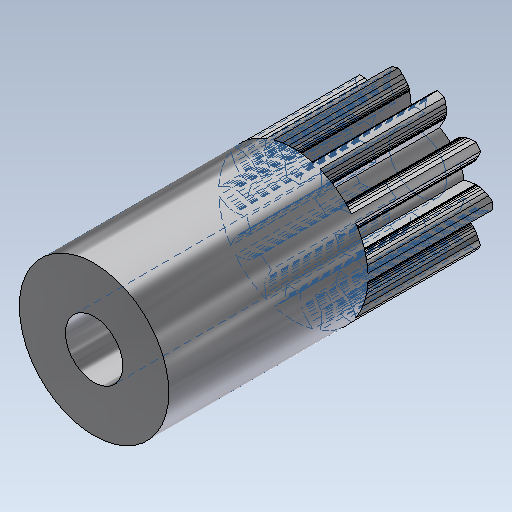
# Autodesk Inventor part: ピニオン10
Saved by Autodesk Inventor 2020 (Build 240168000, 168)
## iProperties
Created: 2015-02-03
Part Number: ピニオン10
Material: 鋼、炭素鋼
Document SubType Name: Modeling
Designer: Riku
Mass: 5 g
Surface Area: 4.55834 cm^2
Volume: 0.265293 cm^3
Density: 18.8471 g/cm^3
Appearance: 半つや出し
Author: Riku
Autodesk Inventor part; units mm, degrees
ref_plane "YZ Plane" through (0, 0, 0) normal (1, 0, 0) x (0, 1, 0)
ref_plane "XZ Plane" through (0, 0, 0) normal (0, 1, 0) x (-1, 0, 0)
ref_plane "XY Plane" through (0, 0, 0) normal (0, 0, 1) x (1, 0, 0)
sketch "スケッチ1" plane through (0, 0, 0) normal (0, 0, 1) x (1, 0, 0)
  arc A0 (148.8341, 107.332) -> (148.8329, 107.3255) centre (148.9303, 107.3099) ccw
  line L0 (148.8329, 107.3255) -> (148.7657, 106.8561)
  arc A1 (148.7657, 106.8561) -> (148.2343, 106.8561) centre (148.5, 105) ccw
  line L1 (148.2343, 106.8561) -> (148.1671, 107.3255)
  arc A2 (148.1671, 107.3255) -> (148.1659, 107.332) centre (148.0697, 107.3099) ccw
  arc A3 (148.1659, 107.332) -> (148.1608, 107.3513) centre (147.9057, 107.2734) ccw
  arc A4 (148.1608, 107.3513) -> (148.1495, 107.3837) centre (147.7349, 107.2218) ccw
  arc A5 (148.1495, 107.3837) -> (148.1294, 107.4297) centre (147.5632, 107.155) ccw
  arc A6 (148.1294, 107.4297) -> (148.0969, 107.4902) centre (147.3904, 107.0715) ccw
  arc A7 (148.0969, 107.4902) -> (148.0472, 107.5661) centre (147.2163, 106.9684) ccw
  arc A8 (148.0472, 107.5661) -> (147.9738, 107.6586) centre (147.0409, 106.8423) ccw
  arc A9 (147.9738, 107.6586) -> (147.8671, 107.7684) centre (146.865, 106.6883) ccw
  arc A10 (147.8671, 107.7684) -> (147.7137, 107.8951) centre (146.6903, 106.5) ccw
  arc A11 (147.7137, 107.8951) -> (147.4344, 107.8044) centre (148.5, 105) ccw
  arc A12 (147.4344, 107.8044) -> (147.3848, 107.6117) centre (149.0824, 107.2772) ccw
  arc A13 (147.3848, 107.6117) -> (147.363, 107.4602) centre (148.8304, 107.327) ccw
  arc A14 (147.363, 107.4602) -> (147.358, 107.3422) centre (148.5975, 107.3481) ccw
  arc A15 (147.358, 107.3422) -> (147.3624, 107.2515) centre (148.3815, 107.347) ccw
  arc A16 (147.3624, 107.2515) -> (147.3717, 107.1835) centre (148.1801, 107.328) ccw
  arc A17 (147.3717, 107.1835) -> (147.3825, 107.1344) centre (147.9912, 107.2941) ccw
  arc A18 (147.3825, 107.1344) -> (147.3924, 107.1016) centre (147.8131, 107.2472) ccw
  arc A19 (147.3924, 107.1016) -> (147.3996, 107.083) centre (147.6446, 107.1885) ccw
  arc A20 (147.3996, 107.083) -> (147.4024, 107.0771) centre (147.4904, 107.1217) ccw
  line L2 (147.4024, 107.0771) -> (147.624, 106.6578)
  arc A21 (147.624, 106.6578) -> (147.1941, 106.3454) centre (148.5, 105) ccw
  line L3 (147.1941, 106.3454) -> (146.8638, 106.6857)
  arc A22 (146.8638, 106.6857) -> (146.859, 106.6902) centre (146.7941, 106.6158) ccw
  arc A23 (146.859, 106.6902) -> (146.8435, 106.7028) centre (146.6829, 106.4899) ccw
  arc A24 (146.8435, 106.7028) -> (146.8154, 106.7224) centre (146.5751, 106.3477) ccw
  arc A25 (146.8154, 106.7224) -> (146.7721, 106.7478) centre (146.4754, 106.1928) ccw
  arc A26 (146.7721, 106.7478) -> (146.7102, 106.7777) centre (146.3848, 106.0237) ccw
  arc A27 (146.7102, 106.7777) -> (146.6254, 106.8099) centre (146.3045, 105.838) ccw
  arc A28 (146.6254, 106.8099) -> (146.5115, 106.8416) centre (146.2367, 105.6329) ccw
  arc A29 (146.5115, 106.8416) -> (146.3608, 106.8677) centre (146.1848, 105.4048) ccw
  arc A30 (146.3608, 106.8677) -> (146.1622, 106.8801) centre (146.1542, 105.1498) ccw
  arc A31 (146.1622, 106.8801) -> (145.9895, 106.6424) centre (148.5, 105) ccw
  arc A32 (145.9895, 106.6424) -> (146.0626, 106.4574) centre (147.6327, 107.1847) ccw
  arc A33 (146.0626, 106.4574) -> (146.1341, 106.3221) centre (147.3995, 107.0767) ccw
  arc A34 (146.1341, 106.3221) -> (146.1994, 106.2236) centre (147.1987, 106.957) ccw
  arc A35 (146.1994, 106.2236) -> (146.2563, 106.1529) centre (147.0246, 106.8291) ccw
  arc A36 (146.2563, 106.1529) -> (146.3037, 106.1032) centre (146.8728, 106.6954) ccw
  arc A37 (146.3037, 106.1032) -> (146.3413, 106.0699) centre (146.7399, 106.5569) ccw
  arc A38 (146.3413, 106.0699) -> (146.3686, 106.0492) centre (146.6234, 106.4142) ccw
  arc A39 (146.3686, 106.0492) -> (146.3854, 106.0384) centre (146.5216, 106.2678) ccw
  arc A40 (146.3854, 106.0384) -> (146.3912, 106.0352) centre (146.4361, 106.1231) ccw
  line L4 (146.3912, 106.0352) -> (146.8169, 105.8262)
  arc A41 (146.8169, 105.8262) -> (146.6527, 105.3209) centre (148.5, 105) ccw
  line L5 (146.6527, 105.3209) -> (146.1854, 105.402)
  arc A42 (146.1854, 105.402) -> (146.1789, 105.4028) centre (146.1702, 105.3045) ccw
  arc A43 (146.1789, 105.4028) -> (146.159, 105.4039) centre (146.1542, 105.1373) ccw
  arc A44 (146.159, 105.4039) -> (146.1247, 105.4033) centre (146.1505, 104.9589) ccw
  arc A45 (146.1247, 105.4033) -> (146.0747, 105.3984) centre (146.1609, 104.775) ccw
  arc A46 (146.0747, 105.3984) -> (146.0071, 105.3862) centre (146.187, 104.5849) ccw
  arc A47 (146.0071, 105.3862) -> (145.9195, 105.3624) centre (146.2312, 104.3874) ccw
  arc A48 (145.9195, 105.3624) -> (145.8089, 105.3211) centre (146.297, 104.1816) ccw
  arc A49 (145.8089, 105.3211) -> (145.6715, 105.2536) centre (146.389, 103.9667) ccw
  arc A50 (145.6715, 105.2536) -> (145.5036, 105.1469) centre (146.5142, 103.7424) ccw
  arc A51 (145.5036, 105.1469) -> (145.5036, 104.8531) centre (148.5, 105) ccw
  arc A52 (145.5036, 104.8531) -> (145.6715, 104.7464) centre (146.5142, 106.2576) ccw
  arc A53 (145.6715, 104.7464) -> (145.8089, 104.6789) centre (146.389, 106.0333) ccw
  arc A54 (145.8089, 104.6789) -> (145.9195, 104.6376) centre (146.297, 105.8184) ccw
  arc A55 (145.9195, 104.6376) -> (146.0071, 104.6138) centre (146.2312, 105.6126) ccw
  arc A56 (146.0071, 104.6138) -> (146.0747, 104.6016) centre (146.187, 105.4151) ccw
  arc A57 (146.0747, 104.6016) -> (146.1247, 104.5967) centre (146.1609, 105.225) ccw
  arc A58 (146.1247, 104.5967) -> (146.159, 104.5961) centre (146.1505, 105.0411) ccw
  arc A59 (146.159, 104.5961) -> (146.1789, 104.5972) centre (146.1542, 104.8627) ccw
  arc A60 (146.1789, 104.5972) -> (146.1854, 104.598) centre (146.1702, 104.6955) ccw
  line L6 (146.1854, 104.598) -> (146.6527, 104.6791)
  arc A61 (146.6527, 104.6791) -> (146.8169, 104.1738) centre (148.5, 105) ccw
  line L7 (146.8169, 104.1738) -> (146.3912, 103.9648)
  arc A62 (146.3912, 103.9648) -> (146.3854, 103.9616) centre (146.4361, 103.8769) ccw
  arc A63 (146.3854, 103.9616) -> (146.3686, 103.9508) centre (146.5216, 103.7322) ccw
  arc A64 (146.3686, 103.9508) -> (146.3413, 103.9301) centre (146.6234, 103.5858) ccw
  arc A65 (146.3413, 103.9301) -> (146.3037, 103.8968) centre (146.7399, 103.4431) ccw
  arc A66 (146.3037, 103.8968) -> (146.2563, 103.8471) centre (146.8728, 103.3046) ccw
  arc A67 (146.2563, 103.8471) -> (146.1994, 103.7764) centre (147.0246, 103.1709) ccw
  arc A68 (146.1994, 103.7764) -> (146.1341, 103.6779) centre (147.1987, 103.043) ccw
  arc A69 (146.1341, 103.6779) -> (146.0626, 103.5426) centre (147.3995, 102.9233) ccw
  arc A70 (146.0626, 103.5426) -> (145.9895, 103.3576) centre (147.6327, 102.8153) ccw
  arc A71 (145.9895, 103.3576) -> (146.1622, 103.1199) centre (148.5, 105) ccw
  arc A72 (146.1622, 103.1199) -> (146.3608, 103.1323) centre (146.1542, 104.8502) ccw
  arc A73 (146.3608, 103.1323) -> (146.5115, 103.1584) centre (146.1848, 104.5952) ccw
  arc A74 (146.5115, 103.1584) -> (146.6254, 103.1901) centre (146.2367, 104.3671) ccw
  arc A75 (146.6254, 103.1901) -> (146.7102, 103.2223) centre (146.3045, 104.162) ccw
  arc A76 (146.7102, 103.2223) -> (146.7721, 103.2522) centre (146.3848, 103.9763) ccw
  arc A77 (146.7721, 103.2522) -> (146.8154, 103.2776) centre (146.4754, 103.8072) ccw
  arc A78 (146.8154, 103.2776) -> (146.8435, 103.2972) centre (146.5751, 103.6523) ccw
  arc A79 (146.8435, 103.2972) -> (146.859, 103.3098) centre (146.6829, 103.5101) ccw
  arc A80 (146.859, 103.3098) -> (146.8638, 103.3143) centre (146.7941, 103.3842) ccw
  line L8 (146.8638, 103.3143) -> (147.1941, 103.6546)
  arc A81 (147.1941, 103.6546) -> (147.624, 103.3422) centre (148.5, 105) ccw
  line L9 (147.624, 103.3422) -> (147.4024, 102.9229)
  arc A82 (147.4024, 102.9229) -> (147.3996, 102.917) centre (147.4904, 102.8783) ccw
  arc A83 (147.3996, 102.917) -> (147.3924, 102.8984) centre (147.6446, 102.8115) ccw
  arc A84 (147.3924, 102.8984) -> (147.3825, 102.8656) centre (147.8131, 102.7528) ccw
  arc A85 (147.3825, 102.8656) -> (147.3717, 102.8165) centre (147.9912, 102.7059) ccw
  arc A86 (147.3717, 102.8165) -> (147.3624, 102.7485) centre (148.1801, 102.672) ccw
  arc A87 (147.3624, 102.7485) -> (147.358, 102.6578) centre (148.3815, 102.653) ccw
  arc A88 (147.358, 102.6578) -> (147.363, 102.5398) centre (148.5975, 102.6519) ccw
  arc A89 (147.363, 102.5398) -> (147.3848, 102.3883) centre (148.8304, 102.673) ccw
  arc A90 (147.3848, 102.3883) -> (147.4344, 102.1956) centre (149.0824, 102.7228) ccw
  arc A91 (147.4344, 102.1956) -> (147.7137, 102.1049) centre (148.5, 105) ccw
  arc A92 (147.7137, 102.1049) -> (147.8671, 102.2316) centre (146.6903, 103.5) ccw
  arc A93 (147.8671, 102.2316) -> (147.9738, 102.3414) centre (146.865, 103.3117) ccw
  arc A94 (147.9738, 102.3414) -> (148.0472, 102.4339) centre (147.0409, 103.1577) ccw
  arc A95 (148.0472, 102.4339) -> (148.0969, 102.5098) centre (147.2163, 103.0316) ccw
  arc A96 (148.0969, 102.5098) -> (148.1294, 102.5703) centre (147.3904, 102.9285) ccw
  arc A97 (148.1294, 102.5703) -> (148.1495, 102.6163) centre (147.5632, 102.845) ccw
  arc A98 (148.1495, 102.6163) -> (148.1608, 102.6487) centre (147.7349, 102.7782) ccw
  arc A99 (148.1608, 102.6487) -> (148.1659, 102.668) centre (147.9057, 102.7266) ccw
  arc A100 (148.1659, 102.668) -> (148.1671, 102.6745) centre (148.0697, 102.6901) ccw
  line L10 (148.1671, 102.6745) -> (148.2343, 103.1439)
  arc A101 (148.2343, 103.1439) -> (148.7657, 103.1439) centre (148.5, 105) ccw
  line L11 (148.7657, 103.1439) -> (148.8329, 102.6745)
  arc A102 (148.8329, 102.6745) -> (148.8341, 102.668) centre (148.9303, 102.6901) ccw
  arc A103 (148.8341, 102.668) -> (148.8392, 102.6487) centre (149.0943, 102.7266) ccw
  arc A104 (148.8392, 102.6487) -> (148.8505, 102.6163) centre (149.2651, 102.7782) ccw
  arc A105 (148.8505, 102.6163) -> (148.8706, 102.5703) centre (149.4368, 102.845) ccw
  arc A106 (148.8706, 102.5703) -> (148.9031, 102.5098) centre (149.6096, 102.9285) ccw
  arc A107 (148.9031, 102.5098) -> (148.9528, 102.4339) centre (149.7837, 103.0316) ccw
  arc A108 (148.9528, 102.4339) -> (149.0262, 102.3414) centre (149.9591, 103.1577) ccw
  arc A109 (149.0262, 102.3414) -> (149.1329, 102.2316) centre (150.135, 103.3117) ccw
  arc A110 (149.1329, 102.2316) -> (149.2863, 102.1049) centre (150.3097, 103.5) ccw
  arc A111 (149.2863, 102.1049) -> (149.5656, 102.1956) centre (148.5, 105) ccw
  arc A112 (149.5656, 102.1956) -> (149.6152, 102.3883) centre (147.9176, 102.7228) ccw
  arc A113 (149.6152, 102.3883) -> (149.637, 102.5398) centre (148.1696, 102.673) ccw
  arc A114 (149.637, 102.5398) -> (149.642, 102.6578) centre (148.4025, 102.6519) ccw
  arc A115 (149.642, 102.6578) -> (149.6376, 102.7485) centre (148.6185, 102.653) ccw
  arc A116 (149.6376, 102.7485) -> (149.6283, 102.8165) centre (148.8199, 102.672) ccw
  arc A117 (149.6283, 102.8165) -> (149.6175, 102.8656) centre (149.0088, 102.7059) ccw
  arc A118 (149.6175, 102.8656) -> (149.6076, 102.8984) centre (149.1869, 102.7528) ccw
  arc A119 (149.6076, 102.8984) -> (149.6004, 102.917) centre (149.3554, 102.8115) ccw
  arc A120 (149.6004, 102.917) -> (149.5976, 102.9229) centre (149.5096, 102.8783) ccw
  line L12 (149.5976, 102.9229) -> (149.376, 103.3422)
  arc A121 (149.376, 103.3422) -> (149.8059, 103.6546) centre (148.5, 105) ccw
  line L13 (149.8059, 103.6546) -> (150.1362, 103.3143)
  arc A122 (150.1362, 103.3143) -> (150.141, 103.3098) centre (150.2059, 103.3842) ccw
  arc A123 (150.141, 103.3098) -> (150.1565, 103.2972) centre (150.3171, 103.5101) ccw
  arc A124 (150.1565, 103.2972) -> (150.1846, 103.2776) centre (150.4249, 103.6523) ccw
  arc A125 (150.1846, 103.2776) -> (150.2279, 103.2522) centre (150.5246, 103.8072) ccw
  arc A126 (150.2279, 103.2522) -> (150.2898, 103.2223) centre (150.6152, 103.9763) ccw
  arc A127 (150.2898, 103.2223) -> (150.3746, 103.1901) centre (150.6955, 104.162) ccw
  arc A128 (150.3746, 103.1901) -> (150.4885, 103.1584) centre (150.7633, 104.3671) ccw
  arc A129 (150.4885, 103.1584) -> (150.6392, 103.1323) centre (150.8152, 104.5952) ccw
  arc A130 (150.6392, 103.1323) -> (150.8378, 103.1199) centre (150.8458, 104.8502) ccw
  arc A131 (150.8378, 103.1199) -> (151.0105, 103.3576) centre (148.5, 105) ccw
  arc A132 (151.0105, 103.3576) -> (150.9374, 103.5426) centre (149.3673, 102.8153) ccw
  arc A133 (150.9374, 103.5426) -> (150.8659, 103.6779) centre (149.6005, 102.9233) ccw
  arc A134 (150.8659, 103.6779) -> (150.8006, 103.7764) centre (149.8013, 103.043) ccw
  arc A135 (150.8006, 103.7764) -> (150.7437, 103.8471) centre (149.9754, 103.1709) ccw
  arc A136 (150.7437, 103.8471) -> (150.6963, 103.8968) centre (150.1272, 103.3046) ccw
  arc A137 (150.6963, 103.8968) -> (150.6587, 103.9301) centre (150.2601, 103.4431) ccw
  arc A138 (150.6587, 103.9301) -> (150.6314, 103.9508) centre (150.3766, 103.5858) ccw
  arc A139 (150.6314, 103.9508) -> (150.6146, 103.9616) centre (150.4784, 103.7322) ccw
  arc A140 (150.6146, 103.9616) -> (150.6088, 103.9648) centre (150.5639, 103.8769) ccw
  line L14 (150.6088, 103.9648) -> (150.1831, 104.1738)
  arc A141 (150.1831, 104.1738) -> (150.3473, 104.6791) centre (148.5, 105) ccw
  line L15 (150.3473, 104.6791) -> (150.8146, 104.598)
  arc A142 (150.8146, 104.598) -> (150.8211, 104.5972) centre (150.8298, 104.6955) ccw
  arc A143 (150.8211, 104.5972) -> (150.841, 104.5961) centre (150.8458, 104.8627) ccw
  arc A144 (150.841, 104.5961) -> (150.8753, 104.5967) centre (150.8495, 105.0411) ccw
  arc A145 (150.8753, 104.5967) -> (150.9253, 104.6016) centre (150.8391, 105.225) ccw
  arc A146 (150.9253, 104.6016) -> (150.9929, 104.6138) centre (150.813, 105.4151) ccw
  arc A147 (150.9929, 104.6138) -> (151.0805, 104.6376) centre (150.7688, 105.6126) ccw
  arc A148 (151.0805, 104.6376) -> (151.1911, 104.6789) centre (150.703, 105.8184) ccw
  arc A149 (151.1911, 104.6789) -> (151.3285, 104.7464) centre (150.611, 106.0333) ccw
  arc A150 (151.3285, 104.7464) -> (151.4964, 104.8531) centre (150.4858, 106.2576) ccw
  arc A151 (151.4964, 104.8531) -> (151.4964, 105.1469) centre (148.5, 105) ccw
  arc A152 (151.4964, 105.1469) -> (151.3285, 105.2536) centre (150.4858, 103.7424) ccw
  arc A153 (151.3285, 105.2536) -> (151.1911, 105.3211) centre (150.611, 103.9667) ccw
  arc A154 (151.1911, 105.3211) -> (151.0805, 105.3624) centre (150.703, 104.1816) ccw
  arc A155 (151.0805, 105.3624) -> (150.9929, 105.3862) centre (150.7688, 104.3874) ccw
  arc A156 (150.9929, 105.3862) -> (150.9253, 105.3984) centre (150.813, 104.5849) ccw
  arc A157 (150.9253, 105.3984) -> (150.8753, 105.4033) centre (150.8391, 104.775) ccw
  arc A158 (150.8753, 105.4033) -> (150.841, 105.4039) centre (150.8495, 104.9589) ccw
  arc A159 (150.841, 105.4039) -> (150.8211, 105.4028) centre (150.8458, 105.1373) ccw
  arc A160 (150.8211, 105.4028) -> (150.8146, 105.402) centre (150.8298, 105.3045) ccw
  line L16 (150.8146, 105.402) -> (150.3473, 105.3209)
  arc A161 (150.3473, 105.3209) -> (150.1831, 105.8262) centre (148.5, 105) ccw
  line L17 (150.1831, 105.8262) -> (150.6088, 106.0352)
  arc A162 (150.6088, 106.0352) -> (150.6146, 106.0384) centre (150.5639, 106.1231) ccw
  arc A163 (150.6146, 106.0384) -> (150.6314, 106.0492) centre (150.4784, 106.2678) ccw
  arc A164 (150.6314, 106.0492) -> (150.6587, 106.0699) centre (150.3766, 106.4142) ccw
  arc A165 (150.6587, 106.0699) -> (150.6963, 106.1032) centre (150.2601, 106.5569) ccw
  arc A166 (150.6963, 106.1032) -> (150.7437, 106.1529) centre (150.1272, 106.6954) ccw
  arc A167 (150.7437, 106.1529) -> (150.8006, 106.2236) centre (149.9754, 106.8291) ccw
  arc A168 (150.8006, 106.2236) -> (150.8659, 106.3221) centre (149.8013, 106.957) ccw
  arc A169 (150.8659, 106.3221) -> (150.9374, 106.4574) centre (149.6005, 107.0767) ccw
  arc A170 (150.9374, 106.4574) -> (151.0105, 106.6424) centre (149.3673, 107.1847) ccw
  arc A171 (151.0105, 106.6424) -> (150.8378, 106.8801) centre (148.5, 105) ccw
  arc A172 (150.8378, 106.8801) -> (150.6392, 106.8677) centre (150.8458, 105.1498) ccw
  arc A173 (150.6392, 106.8677) -> (150.4885, 106.8416) centre (150.8152, 105.4048) ccw
  arc A174 (150.4885, 106.8416) -> (150.3746, 106.8099) centre (150.7633, 105.6329) ccw
  arc A175 (150.3746, 106.8099) -> (150.2898, 106.7777) centre (150.6955, 105.838) ccw
  arc A176 (150.2898, 106.7777) -> (150.2279, 106.7478) centre (150.6152, 106.0237) ccw
  arc A177 (150.2279, 106.7478) -> (150.1846, 106.7224) centre (150.5246, 106.1928) ccw
  arc A178 (150.1846, 106.7224) -> (150.1565, 106.7028) centre (150.4249, 106.3477) ccw
  arc A179 (150.1565, 106.7028) -> (150.141, 106.6902) centre (150.3171, 106.4899) ccw
  arc A180 (150.141, 106.6902) -> (150.1362, 106.6857) centre (150.2059, 106.6158) ccw
  line L18 (150.1362, 106.6857) -> (149.8059, 106.3454)
  arc A181 (149.8059, 106.3454) -> (149.376, 106.6578) centre (148.5, 105) ccw
  line L19 (149.376, 106.6578) -> (149.5976, 107.0771)
  arc A182 (149.5976, 107.0771) -> (149.6004, 107.083) centre (149.5096, 107.1217) ccw
  arc A183 (149.6004, 107.083) -> (149.6076, 107.1016) centre (149.3554, 107.1885) ccw
  arc A184 (149.6076, 107.1016) -> (149.6175, 107.1344) centre (149.1869, 107.2472) ccw
  arc A185 (149.6175, 107.1344) -> (149.6283, 107.1835) centre (149.0088, 107.2941) ccw
  arc A186 (149.6283, 107.1835) -> (149.6376, 107.2515) centre (148.8199, 107.328) ccw
  arc A187 (149.6376, 107.2515) -> (149.642, 107.3422) centre (148.6185, 107.347) ccw
  arc A188 (149.642, 107.3422) -> (149.637, 107.4602) centre (148.4025, 107.3481) ccw
  arc A189 (149.637, 107.4602) -> (149.6152, 107.6117) centre (148.1696, 107.327) ccw
  arc A190 (149.6152, 107.6117) -> (149.5656, 107.8044) centre (147.9176, 107.2772) ccw
  arc A191 (149.5656, 107.8044) -> (149.2863, 107.8951) centre (148.5, 105) ccw
  arc A192 (149.2863, 107.8951) -> (149.1329, 107.7684) centre (150.3097, 106.5) ccw
  arc A193 (149.1329, 107.7684) -> (149.0262, 107.6586) centre (150.135, 106.6883) ccw
  arc A194 (149.0262, 107.6586) -> (148.9528, 107.5661) centre (149.9591, 106.8423) ccw
  arc A195 (148.9528, 107.5661) -> (148.9031, 107.4902) centre (149.7837, 106.9684) ccw
  arc A196 (148.9031, 107.4902) -> (148.8706, 107.4297) centre (149.6096, 107.0715) ccw
  arc A197 (148.8706, 107.4297) -> (148.8505, 107.3837) centre (149.4368, 107.155) ccw
  arc A198 (148.8505, 107.3837) -> (148.8392, 107.3513) centre (149.2651, 107.2218) ccw
  arc A199 (148.8392, 107.3513) -> (148.8341, 107.332) centre (149.0943, 107.2734) ccw
  circle A200 centre (148.5, 105) radius 1.15
  point P0 (0, 0)
  point P1 (225, 22)
  point P2 (225, 14)
  dimension "d0" = 2.3
  constraints: 400 point on circle, 201 centre point, 40 end point, 1 coincident, 2 other
  measures "d0" diameter of A200
extrude "押し出し1" add sketch "スケッチ1" along normal blind 5
sketch "スケッチ2" plane through (0, 0, 5) normal (0, 0, 1) x (1, 0, 0)
  circle A0 centre (148.5, 105) radius 1.15 projected
  circle A1 centre (148.5, 105) radius 3
  point P0 (0, 0)
  dimension "d3" = 6
  constraints: 1 centre point, 1 coincident
  measures "d3" diameter of A1
extrude "押し出し2" add sketch "スケッチ2" along normal blind 8
